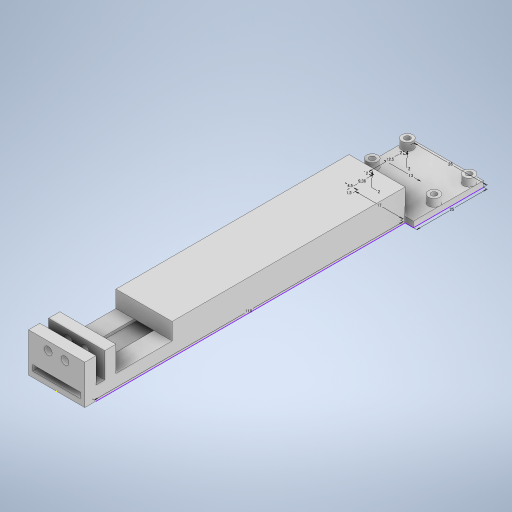
# Autodesk Inventor part: MouthCameraBase
Saved by Autodesk Inventor 2024.2 (Build 282272000, 272)
## iProperties
Created: 2024-04-06
Part Number: MouthCameraBase
Material: 一般
Document SubType Name: Modeling
Designer: yukin
Density: 1 g/cm^3
Appearance: 既定
Author: yukin
Autodesk Inventor part; units mm, degrees
ref_plane "YZ Plane" through (0, 0, 0) normal (1, 0, 0) x (0, 1, 0)
ref_plane "XZ Plane" through (0, 0, 0) normal (0, 1, 0) x (-1, 0, 0)
ref_plane "XY Plane" through (0, 0, 0) normal (0, 0, 1) x (1, 0, 0)
sketch "スケッチ1" plane through (0, 0, 0) normal (0, 1, 0) x (-1, 0, 0)
  line L0 (8.5, 24.0956) -> (-8.5, 24.0956)
  line L1 (-8.5, 24.0956) -> (-8.5, -85.9044)
  line L2 (-8.5, -85.9044) -> (8.5, -85.9044)
  line L3 (8.5, -85.9044) -> (8.5, 24.0956)
  line L4 (13, -85.9044) -> (-13, -85.9044)
  line L5 (-13, -85.9044) -> (-13, -110.9044)
  line L6 (-13, -110.9044) -> (13, -110.9044)
  line L7 (13, -110.9044) -> (13, -85.9044)
  circle A0 centre (11, -95.2644) radius 1
  circle A1 centre (11, -107.7644) radius 1
  line L8 (0, -85.9044) -> (0, -110.9044)
  line L9 (-8.5, -85.9044) -> (-8.5, 24.0956)
  circle A2 centre (-11, -95.2644) radius 1
  circle A3 centre (-11, -107.7644) radius 1
  line L10 (0, -85.9044) -> (0, 24.0956)
  line L11 (10, -85.9044) -> (10, 24.0956)
  line L12 (10, 24.0956) -> (8.5, 24.0956)
  line L13 (-8.5, -85.9044) -> (-8.5, 24.0956)
  line L14 (-10, -85.9044) -> (-10, 24.0956)
  line L15 (-10, 24.0956) -> (-8.5, 24.0956)
  line L16 (10, 24.0956) -> (-10, 24.0956)
  line L17 (8.5, 24.0956) -> (-8.5, 24.0956)
  line L18 (10, 24.0956) -> (-10, 24.0956)
  point P0 (0, 0)
  point P1 (-8.5, 24.0956)
  dimension "d0" = 17
  dimension "d1" = 110
  dimension "d2" = 26
  dimension "d3" = 25
  dimension "d4" = 4.5
  dimension "d5" = 2
  dimension "d6" = 9.36
  dimension "d7" = 2
  dimension "d8" = 12.5
  dimension "d9" = 2
  dimension "d10" = 2
  dimension "d11" = 13
  dimension "d12" = 1.5
  constraints: 38 end point, 6 equal length, 6 symmetric about line, 4 centre point, 4 horizontal, 4 perpendicular, 3 midpoint, 2 point on line, 2 other
  measures "d0" distance of L2.end L1.end
  measures "d1" distance of L1.end L0.end
  measures "d2" distance of L6.end L5.end
  measures "d3" distance of L5.end L4.end
  measures "d4" distance between parallel lines of L7 L3
  measures "d5" diameter of A0
  measures "d6" distance from line of A0.centre L4
  measures "d7" diameter of A1
  measures "d8" distance of A1.centre A0.centre
  measures "d9" distance from line of L7 A0.centre
  measures "d10" distance from line of L7 A1.centre
  measures "d11" distance between parallel lines of L8 L7
  measures "d12" distance between parallel lines of L3 L11
extrude "押し出し1" add sketch "スケッチ1" along normal blind 2 contours L3 L2 L10 L0 | L10 L2 L1 L0 | L4 L7 L6 L8 L2 | L8 L6 L5 L4 L2
extrude "押し出し2" add sketch "スケッチ1" along normal blind 5 contours L12 L11 L4 L3 | L1 L4 L14 L15
sketch "スケッチ2" plane through (-8.5, 2, 24.0956) normal (1, 0, 0) x (0, 0, -1)
  line L0 (0, 0) -> (0, 3) projected
  line L1 (0, 3) -> (110, 3)
  line L2 (110, 3) -> (110, 2)
  line L3 (110, 2) -> (0, 2)
  line L4 (0, 2) -> (0, 3)
  point P0 (24.0956, -2)
  point P1 (0, 2)
  dimension "d27" = 110
  dimension "d28" = 1
  constraints: 8 end point, 2 parallel, 1 horizontal, 1 perpendicular
  measures "d27" distance of L2.end L3.end
  measures "d28" distance of L1.end L2.end
sketch "スケッチ3" plane through (8.5, 2, -85.9044) normal (-1, 0, 0) x (0, 0, 1)
  line L0 (0, 3) -> (110, 3) projected
  line L1 (0, 3) -> (110, 3)
  line L2 (110, 3) -> (110, 2)
  line L3 (110, 2) -> (0, 2)
  line L4 (0, 2) -> (0, 3)
  point P0 (85.9044, -2)
  dimension "d29" = 110
  dimension "d30" = 1
  constraints: 8 end point, 2 parallel, 1 horizontal, 1 perpendicular
  measures "d29" distance of L2.end L3.end
  measures "d30" distance of L1.end L2.end
sketch "スケッチ5" plane through (-10, 0, 24.0956) normal (0, 0, 1) x (1, 0, 0)
  line L0 (0, 0) -> (0, 2) projected
  line L1 (0, 0) -> (20, 0)
  line L2 (20, 0) -> (20, 14)
  line L3 (20, 14) -> (0, 14)
  line L4 (0, 14) -> (0, 0)
  line L5 (0, 2) -> (1.5, 2) projected
  line L6 (18.5, 4) -> (13.5, 4) projected
  line L7 (1.5, 2) -> (18.5, 2)
  line L8 (18.5, 2) -> (18.5, 4)
  line L9 (18.5, 4) -> (1.5, 4)
  line L10 (1.5, 4) -> (1.5, 2)
  circle A0 centre (7, 11) radius 1.375
  circle A1 centre (13, 11) radius 1.375
  point P0 (10, 0)
  point P1 (0, 2)
  dimension "d35" = 20
  dimension "d36" = 14
  dimension "d37" = 2.75
  dimension "d38" = 2.75
  dimension "d39" = 3
  dimension "d40" = 3
  dimension "d41" = 6
  dimension "d42" = 7
  constraints: 16 end point, 4 parallel, 2 centre point, 2 horizontal, 2 perpendicular
  measures "d35" distance of L3.end L2.end
  measures "d36" distance of L2.end L1.end
  measures "d37" diameter of A0
  measures "d38" diameter of A1
  measures "d39" distance from line of L3 A0.centre
  measures "d40" distance from line of L3 A1.centre
  measures "d41" distance of A1.centre A0.centre
  measures "d42" distance from line of L4 A0.centre
extrude "押し出し5" add sketch "スケッチ5" along normal blind 4
extrude "押し出し6" add sketch "スケッチ2" along normal blind 5
extrude "押し出し7" add sketch "スケッチ3" along normal blind 5
sketch "スケッチ6" plane through (-10, 0, 28.0956) normal (0, 0, 1) x (1, 0, 0)
  point P0 (10, 0)
sketch "スケッチ8" plane through (0, 2, 0) normal (0, 1, 0) x (1, 0, 0)
  circle A0 centre (11, 107.7644) radius 1 projected
  circle A1 centre (11, 107.7644) radius 2
  circle A2 centre (-11, 107.7644) radius 1 projected
  circle A3 centre (-11, 107.7644) radius 2
  circle A4 centre (-11, 95.2644) radius 1 projected
  circle A5 centre (-11, 95.2644) radius 2
  circle A6 centre (11, 95.2644) radius 2
  point P0 (0, 0)
  dimension "d49" = 4
  dimension "d50" = 4
  dimension "d53" = 4
  dimension "d54" = 4
  constraints: 4 centre point, 3 coincident
  measures "d49" diameter of A1
  measures "d50" diameter of A3
  measures "d53" diameter of A5
  measures "d54" diameter of A6
extrude "押し出し8" add sketch "スケッチ8" along normal blind 2.7
extrude "押し出し9" cut sketch "スケッチ1" along normal blind 4.8 contours A2
sketch "スケッチ9" plane through (0, 5, 0) normal (0, 1, 0) x (1, 0, 0)
  line L0 (-10, 85.9044) -> (-10, -24.0956) projected
  line L1 (10, -24.0956) -> (10, 85.9044) projected
  line L2 (-10, -20.9956) -> (10, -20.9956)
  line L3 (10, -20.9956) -> (10, -16.9956)
  line L4 (10, -16.9956) -> (-10, -16.9956)
  line L5 (-10, -16.9956) -> (-10, -20.9956)
  line L6 (10, -24.0956) -> (-10, -24.0956) projected
  point P0 (0, 0)
  point P1 (10, -20.9956)
  dimension "d57" = 3.1
  dimension "d58" = 4
  constraints: 8 end point, 2 parallel, 2 point on line, 1 horizontal, 1 perpendicular
  measures "d57" distance between parallel lines of L2 L6
  measures "d58" distance between parallel lines of L4 L2
extrude "押し出し10" add sketch "スケッチ9" along normal blind 9 contours L4 L1 L2 L0
sketch "スケッチ10" plane through (3.5, 5, 16.9956) normal (0, 0, -1) x (-1, 0, 0)
  line L0 (0, 0) -> (-6.5, 0) projected
  line L1 (-6.5, 0) -> (13.5, 0)
  line L2 (13.5, 0) -> (13.5, 6)
  line L3 (13.5, 6) -> (-6.5, 6)
  line L4 (-6.5, 6) -> (-6.5, 0)
  point P0 (3.5, -5)
  dimension "d63" = 20
  dimension "d64" = 6
  constraints: 8 end point, 2 parallel, 1 horizontal, 1 perpendicular
  measures "d63" distance of L3.end L2.end
  measures "d64" distance of L2.end L1.end
extrude "押し出し12" add sketch "スケッチ10" along normal blind 103
extrude "押し出し13" add sketch "スケッチ10" along normal blind 103
extrude "押し出し11" cut sketch "スケッチ5" against normal blind 8 contours A0 | A1
sketch "スケッチ11" plane through (-4.375, 11, 16.9956) normal (0, 1, 0) x (1, 0, 0)
  line L0 (14.375, -11.1) -> (14.375, 102.9) projected
  line L1 (14.375, 0.0015) -> (-5.625, 0.0015)
  line L2 (-5.625, 0.0015) -> (-5.625, 20.0015)
  line L3 (-5.625, 20.0015) -> (14.375, 20.0015)
  line L4 (14.375, 20.0015) -> (14.375, 0.0015)
  point P0 (4.375, 16.9956)
  dimension "d69" = 20
  dimension "d70" = 20
  constraints: 8 end point, 2 parallel, 1 horizontal, 1 perpendicular, 1 point on line
  measures "d69" distance of L2.end L3.end
  measures "d70" distance of L1.end L2.end
extrude "押し出し14" cut sketch "スケッチ11" against normal blind 6
